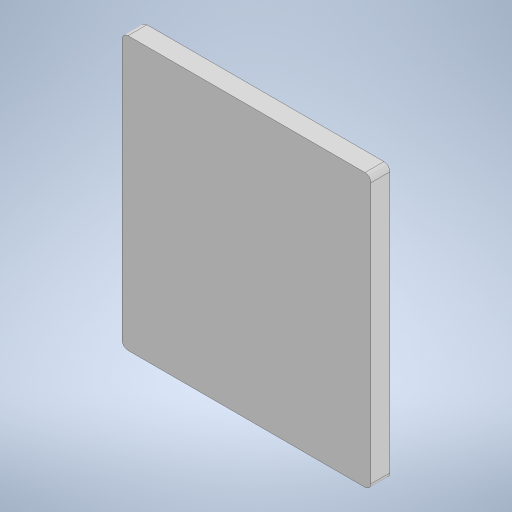
# Autodesk Inventor part: ETH_BRKT_PCB
Saved by Autodesk Inventor 2024.2 (Build 282272000, 272)
## iProperties
Created: 2024-02-23
Part Number: ETH_BRKT_PCB
Material: Generic
Document SubType Name: Modeling
Designer: lgnds
Density: 1 g/cm^3
Appearance: Default
Author: lgnds
Autodesk Inventor part; units mm, degrees
ref_plane "YZ Plane" through (0, 0, 0) normal (1, 0, 0) x (0, 1, 0)
ref_plane "XZ Plane" through (0, 0, 0) normal (0, 1, 0) x (-1, 0, 0)
ref_plane "XY Plane" through (0, 0, 0) normal (0, 0, 1) x (1, 0, 0)
sketch "Sketch1" plane through (0, 0, 0) normal (0, 0, 1) x (1, 0, 0)
  line L0 (-10.5, -11.5) -> (10.5, -11.5)
  line L1 (10.5, -11.5) -> (10.5, 11.5)
  line L2 (10.5, 11.5) -> (-10.5, 11.5)
  line L3 (-10.5, 11.5) -> (-10.5, -11.5)
  line L4 (-10.5, -11.5) -> (10.5, 11.5) construction
  line L5 (10.5, -11.5) -> (-10.5, 11.5) construction
  point P0 (0, 0)
  dimension "d1" = 21
  dimension "d2" = 23
  constraints: 12 end point, 2 midpoint, 2 parallel, 1 horizontal, 1 perpendicular
  measures "d1" distance between parallel lines of L3 L1
  measures "d2" distance between parallel lines of L0 L2
extrude "Extrusion1" add sketch "Sketch1" along normal blind 1.6
fillet "Fillet1" radius 0.5 4 edges at (10.5, 11.5, 0.8) (10.5, -11.5, 0.8) (-10.5, -11.5, 0.8) (-10.5, 11.5, 0.8)
body "Solid1"
